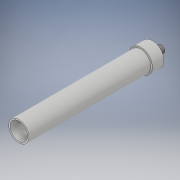
# Autodesk Inventor part: long pipe
Saved by Autodesk Inventor 2018 (Build 220112000, 112)
## iProperties
Created: 2017-05-02
Part Number: long pipe
Material: Generic
Document SubType Name: Modeling
Designer: gsegs
Density: 1 g/cm^3
Appearance: Default
Author: gsegs
Autodesk Inventor part; units mm, degrees
ref_plane "YZ Plane" through (0, 0, 0) normal (1, 0, 0) x (0, 1, 0)
ref_plane "XZ Plane" through (0, 0, 0) normal (0, 1, 0) x (-1, 0, 0)
ref_plane "XY Plane" through (0, 0, 0) normal (0, 0, 1) x (1, 0, 0)
sketch "Sketch1" plane through (0, 0, 0) normal (0, 0, 1) x (1, 0, 0)
  circle A0 centre (-53.0097, 46.3835) radius 44.45
  point P0 (0, 0)
  dimension "d0" = 88.9
  constraints: 1 centre point
  measures "d0" diameter of A0
extrude "Extrusion1" add sketch "Sketch1" along normal blind 584.2
sketch "Sketch2" plane through (-53.0097, 46.3835, 0) normal (0, 0, -1) x (-1, 0, 0)
  circle A0 centre (0, 0) radius 44.45 projected
  circle A1 centre (0, 0) radius 50.5264
  point P0 (-53.0097, -46.3835)
  dimension "d3" = 6.0764
  constraints: 1 centre point
  measures "d3" radial gap between concentric circles of A0 A1
extrude "Extrusion2" add sketch "Sketch2" against normal blind 50.8 contours A0 | A1
sketch "Sketch3" plane through (-53.0097, 46.3835, 584.2) normal (0, 0, 1) x (1, 0, 0)
  circle A0 centre (0, 0) radius 44.45 projected
  circle A1 centre (0, 0) radius 38.354
  point P0 (53.0097, -46.3835)
  dimension "d6" = 6.096
  constraints: 1 centre point
  measures "d6" radial gap between concentric circles of A1 A0
extrude "Extrusion3" cut sketch "Sketch3" against normal blind 581.025 contours A1
sketch "Sketch4" plane through (-53.0097, 46.3835, 0) normal (0, 0, -1) x (-1, 0, 0)
  circle A0 centre (0, 0) radius 16.637
  point P0 (-53.0097, -46.3835)
  dimension "d9" = 33.274
  constraints: 1 centre point
  measures "d9" diameter of A0
extrude "Extrusion4" add sketch "Sketch4" along normal blind 38.1
thread "Thread1" size "1 5/16-8 UN" class "2A" standard "ANSI Unified Screw Threads" full length
body "Solid1"
